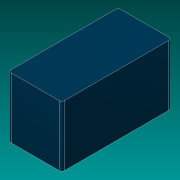
# Autodesk Inventor part: Medio
Saved by Autodesk Inventor 2020.3 (Build 243373000, 373)
## iProperties
Created: 2016-09-26
Part Number: Medio
Material: Aluminum 6061
Document SubType Name: Modeling
Designer: Julian
Density: 2.7 g/cm^3
Appearance: Anodized - Light Gray
Author: Julian
Autodesk Inventor part; units mm, degrees
ref_plane "YZ Plane" through (0, 0, 0) normal (1, 0, 0) x (0, 1, 0)
ref_plane "XZ Plane" through (0, 0, 0) normal (0, 1, 0) x (-1, 0, 0)
ref_plane "XY Plane" through (0, 0, 0) normal (0, 0, 1) x (1, 0, 0)
sketch "Boceto1" plane through (0, 0, 0) normal (0, 1, 0) x (-1, 0, 0)
  line L0 (9.9, 20.3) -> (-9.9, 20.3)
  line L1 (-9.9, 20.3) -> (-9.9, -20.3)
  line L2 (-9.9, -20.3) -> (9.9, -20.3)
  line L3 (9.9, -20.3) -> (9.9, 20.3)
  line L4 (9.9, 20.3) -> (-9.9, -20.3) construction
  line L5 (-9.9, 20.3) -> (9.9, -20.3) construction
  point P0 (0, 0)
  dimension "d0" = 19.8
  dimension "d1" = 40.6
  constraints: 12 end point, 2 midpoint, 2 parallel, 1 horizontal, 1 perpendicular
  measures "d0" distance of L2.end L1.end
  measures "d1" distance of L1.end L0.end
extrude "Extrusión1" add sketch "Boceto1" against normal blind 20.5
fillet "Empalme1" radius 1 4 edges at (9.9, -10.25, 20.3) (-9.9, -10.25, 20.3) (9.9, -10.25, -20.3) (-9.9, -10.25, -20.3)
sketch "Sketch2" plane through (0, 0, 0) normal (0, 1, 0) x (1, 0, 0)
  arc A0 (-8.9, 20.3) -> (-9.9, 19.3) centre (-8.9, 19.3) ccw projected
  line L0 (-9.9, 19.3) -> (-9.9, -19.3) projected
  arc A1 (-9.9, -19.3) -> (-8.9, -20.3) centre (-8.9, -19.3) ccw projected
  line L1 (-8.9, -20.3) -> (8.9, -20.3) projected
  arc A2 (8.9, -20.3) -> (9.9, -19.3) centre (8.9, -19.3) ccw projected
  line L2 (9.9, -19.3) -> (9.9, 19.3) projected
  arc A3 (9.9, 19.3) -> (8.9, 20.3) centre (8.9, 19.3) ccw projected
  line L3 (8.9, 20.3) -> (-8.9, 20.3) projected
  point P0 (0, 0)
extrude "Extrusion2" add sketch "Sketch2" along normal blind 1.9
